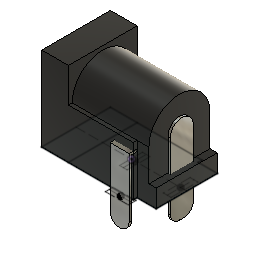
MJ-179PH (Autodesk Fusion 360 design; units mm, degrees)
Autodesk Fusion 360 part; units mm, degrees
sketch "スケッチ1" plane through (0, 0, 0) normal (0, 0, 1) x (1, 0, 0)
  line L0 (-7.25, 4.5) -> (4.75, 4.5)
  line L1 (7.25, 4) -> (7.25, -4)
  line L2 (4.75, -4.5) -> (-7.25, -4.5)
  line L3 (-7.25, -4.5) -> (-7.25, 4.5)
  line L4 (-7.25, 0) -> (7.25, 0) construction
  line L5 (2, -5.4) -> (5, -5.4) construction
  line L6 (5, -5.4) -> (5, -4.4) construction
  line L7 (5, -4.4) -> (2, -4.4) construction
  line L8 (2, -4.4) -> (2, -5.4) construction
  line L9 (-0.05, -1.5) -> (0.95, -1.5) construction
  line L10 (0.95, -1.5) -> (0.95, 1.5) construction
  line L11 (0.95, 1.5) -> (-0.05, 1.5) construction
  line L12 (-0.05, 1.5) -> (-0.05, -1.5) construction
  line L13 (5.95, -1.75) -> (6.95, -1.75) construction
  line L14 (6.95, -1.75) -> (6.95, 1.75) construction
  line L15 (6.95, 1.75) -> (5.95, 1.75) construction
  line L16 (5.95, 1.75) -> (5.95, -1.75) construction
  line L17 (6.45, -1.75) -> (6.45, 1.75) construction
  line L18 (0.45, -1.5) -> (0.45, 1.5) construction
  line L19 (2, -4.9) -> (5, -4.9) construction
  line L20 (4.75, -4.5) -> (4.75, -4)
  line L21 (4.75, -4) -> (7.25, -4)
  line L22 (4.75, 4.5) -> (4.75, 4)
  line L23 (4.75, 4) -> (7.25, 4)
  line L24 (-3.75, -4.5) -> (-3.75, 4.5)
  point P0 (3.5, -4.9)
  point P1 (0.45, 0)
  point P2 (6.45, 0)
  dimension "d2" = 9
  dimension "d3" = 3
  dimension "d4" = 1
  dimension "d5" = 1
  dimension "d6" = 3
  dimension "d7" = 3.5
  dimension "d8" = 1
  dimension "d9" = 7.7
  dimension "d10" = 10.75
  dimension "d11" = 13.7
  dimension "d12" = 4.9
  dimension "d13" = 14.5
  dimension "d14" = 12
  dimension "d15" = 0.5
  dimension "d57" = 3.5
  constraint horizontal L0
  constraint vertical L1
  constraint horizontal L2
  constraint vertical L3
  constraint midpoint L3 L4.start
  constraint midpoint origin L4
  constraint horizontal L5
  constraint vertical L6
  constraint horizontal L7
  constraint vertical L8
  constraint horizontal L9
  constraint vertical L10
  constraint horizontal L11
  constraint vertical L12
  constraint horizontal L13
  constraint vertical L14
  constraint horizontal L15
  constraint vertical L16
  constraint midpoint L13 L17.start
  constraint midpoint L15 L17.end
  constraint midpoint L9 L18.start
  constraint midpoint L11 L18.end
  constraint midpoint L8 L19.start
  constraint midpoint L6 L19.end
  constraint midpoint L19 P0
  constraint midpoint L18 P1
  constraint midpoint L17 P2
  constraint coincident L4 P2
  constraint coincident L4 P1
  constraint perpendicular L2 L20
  constraint perpendicular L1 L21
  constraint perpendicular L0 L22
  constraint perpendicular L1 L23
  constraint coincident L1 L4.end
  constraint midpoint L1 L4.end
  constraint collinear L20 L22
  constraint horizontal L4
  constraint coincident L2 L24.start
  constraint coincident L0 L24.end
  constraint perpendicular L0 L24
  measures "d2" distance of L0.start L2.end
  measures "d3" distance of L5.start L5.end
  measures "d4" distance of L5.start L7.end
  measures "d5" distance of L9.start L9.end
  measures "d6" distance of L9.start L11.end
  measures "d7" distance of L13.end L14.end
  measures "d8" distance of L14.end L15.end
  measures "d9" distance of L3 P1
  measures "d10" distance of L3 P0
  measures "d11" distance of L3 P2
  measures "d12" distance of L4 P0
  measures "d13" distance of L1 L3
  measures "d14" distance of L3 L22
  measures "d15" distance of L0.end L22.end
  measures "d57" distance of L3 L24
sketch "スケッチ3" plane through (0, 0, 0) normal (0, 0, 1) x (1, 0, 0)
  line L0 (2.25, -4.75) -> (4.75, -4.75)
  line L1 (4.75, -4.75) -> (4.75, -5.05)
  line L2 (4.75, -5.05) -> (2.25, -5.05)
  line L3 (2.25, -5.05) -> (2.25, -4.75)
  line L4 (2.25, -4.75) -> (4.75, -5.05) construction
  line L5 (0.3, -1.25) -> (0.3, 1.25)
  line L6 (0.3, 1.25) -> (0.6, 1.25)
  line L7 (0.6, 1.25) -> (0.6, -1.25)
  line L8 (0.6, -1.25) -> (0.3, -1.25)
  line L9 (0.3, 1.25) -> (0.6, -1.25) construction
  line L10 (6.3, -1.5) -> (6.3, 1.5)
  line L11 (6.3, 1.5) -> (6.6, 1.5)
  line L12 (6.6, 1.5) -> (6.6, -1.5)
  line L13 (6.6, -1.5) -> (6.3, -1.5)
  line L14 (6.3, 1.5) -> (6.6, -1.5) construction
  point P0 (3.5, -4.9)
  point P1 (0.45, 0)
  point P2 (6.45, 0)
  dimension "d18" = 2.5
  dimension "d19" = 0.3
  dimension "d20" = 2.5
  dimension "d21" = 0.3
  dimension "d22" = 3
  dimension "d23" = 0.3
  constraint horizontal L0
  constraint vertical L1
  constraint horizontal L2
  constraint vertical L3
  constraint midpoint L4 P0
  constraint midpoint L9 P1
  constraint vertical L5
  constraint horizontal L6
  constraint vertical L7
  constraint horizontal L8
  constraint vertical L10
  constraint horizontal L11
  constraint vertical L12
  constraint horizontal L13
  constraint midpoint L14 P2
  measures "d18" distance of L0.start L0.end
  measures "d19" distance of L0.end L1.end
  measures "d20" distance of L6.end L7.end
  measures "d21" distance of L5.start L7.end
  measures "d22" distance of L11.end L12.end
  measures "d23" distance of L10.start L12.end
sketch "スケッチ5" plane through (0, 0, 0) normal (1, 0, 0) x (0, 1, 0)
  line L0 (4.5, 0) -> (-4.5, 0)
  line L1 (-4.5, 0) -> (-4.5, 11)
  line L2 (-4.5, 11) -> (4.5, 11)
  line L3 (4.5, 11) -> (4.5, 0)
  circle A0 centre (0, 6.5) radius 3
  line L4 (0, 11) -> (0, 0) construction
  circle A1 centre (0, 6.5) radius 0.975
  line L5 (0.975, 6.5) -> (3, 6.5) construction
  circle A2 centre (0, 6.5) radius 1.9875
  line L6 (-1.7319, 5.525) -> (1.7319, 5.525) construction
  point P0 (4.5, 0)
  point P1 (-4.5, 0)
  point P2 (1.9875, 6.5)
  dimension "d26" = 11
  dimension "d27" = 6
  dimension "d28" = 4.5
  dimension "d29" = 9
  dimension "d36" = 1.95
  constraint horizontal L0
  constraint vertical L1
  constraint horizontal L2
  constraint vertical L3
  constraint coincident P0 L0.start
  constraint coincident P1 L0.end
  constraint midpoint L2 L4.start
  constraint coincident L4.end origin
  constraint coincident A0.centre L4
  constraint concentric A0 A1
  constraint coincident A1 L5.start
  constraint coincident A0 L5.end
  constraint horizontal L5
  constraint coincident A0.centre L5
  constraint midpoint L5 P2
  constraint concentric A0 A2
  constraint coincident P2 A2
  constraint coincident A2 L6.start
  constraint coincident A2 L6.end
  constraint perpendicular L4 L6
  constraint tangent A1 L6
  measures "d26" distance of P0 L2.end
  measures "d27" diameter of A0
  measures "d28" distance of L2 A0.centre
  measures "d29" distance of L1.end L2.end
  measures "d36" diameter of A1
sketch "スケッチ4" plane through (0, 0, 0) normal (0, 1, 0) x (1, 0, 0)
  line L0 (-7.25, 0) -> (7.25, 0)
  line L1 (-7.25, 0) -> (-7.25, -11)
  line L2 (-7.25, -11) -> (-3.75, -11)
  line L3 (-3.75, -11) -> (-3.75, -6.5)
  line L4 (-3.75, -6.5) -> (6.3, -6.5)
  line L5 (7.25, 0) -> (7.25, -2.331)
  line L6 (7.25, -2.331) -> (6.3, -2.331)
  line L7 (6.3, -2.331) -> (6.3, -6.5)
  line L8 (4.75, 0) -> (4.75, -6.5)
  line L9 (4.75, -6.5) -> (4.75, -10.5)
  line L10 (4.75, -10.5) -> (-3.75, -10.5)
  line L11 (4.75, -10.5) -> (6.3, -10.5)
  line L12 (6.3, -10.5) -> (6.3, -6.5)
  point P0 (-7.25, 0)
  point P1 (6.3, 0)
  point P2 (4.75, 0)
  point P3 (0, -6.5)
  dimension "d24" = 3.5
  dimension "d25" = 11
  dimension "d30" = 0.5
  constraint coincident P0 L0.start
  constraint perpendicular L0 L1
  constraint perpendicular L1 L2
  constraint perpendicular L2 L3
  constraint perpendicular L3 L4
  constraint coincident L0.end L5.start
  constraint perpendicular L4 L5
  constraint perpendicular L5 L6
  constraint coincident L4 L7.end
  constraint perpendicular L4 L7
  constraint coincident L4.end L7.end
  constraint coincident L7 P1
  constraint coincident P2 L8.start
  constraint coincident L4 L8.end
  constraint perpendicular L4 L8
  constraint coincident L4 P3
  constraint perpendicular L4 L9
  constraint coincident L3 L10.end
  constraint perpendicular L3 L10
  constraint perpendicular L9 L11
  constraint vertical L12
  measures "d24" distance of L1.end L2.end
  measures "d25" distance of P0 L1.end
  measures "d30" distance of L2 L10
extrude "押し出し1" add sketch "スケッチ1" along normal blind 11 makes body 1
extrude "押し出し2" cut sketch "スケッチ4" along normal through all and the other way through all keep common part bodies 1
sketch "スケッチ6" plane through (6.3, 0, 0) normal (1, 0, 0) x (0, 1, 0)
  line L0 (4, 2.331) -> (4, 10.5)
  line L1 (4, 10.5) -> (-4, 10.5)
  line L2 (-4, 10.5) -> (-4, 2.331)
  line L3 (-4, 2.331) -> (4, 2.331)
  arc A0 (4, 6.5) -> (-4, 6.5) centre (0, 6.5) ccw
  line L4 (-4.5, 0) -> (-4.5, 11)
  line L5 (-4, 6.5) -> (-4.5, 6.5)
  line L6 (4.5, 0) -> (4.5, 10.5)
  line L7 (4, 6.5) -> (4.5, 6.5)
  line L8 (-4.5, 0) -> (-4.5, 11)
  line L9 (-4.5, 10.5) -> (-4, 10.5)
  line L10 (-4, 10.5) -> (4, 10.5)
  line L11 (4, 10.5) -> (4.5, 10.5)
  point P0 (0, 6.5)
  point P1 (-4.5, 10.5)
  constraint coincident P0 A0.centre
  constraint tangent L1 A0
  constraint coincident L2 A0.end
  constraint coincident L0 A0.start
  constraint coincident L4 L5.end
  constraint perpendicular L2 L5
  constraint coincident L6 L7.end
  constraint perpendicular L0 L7
extrude "押し出し3" cut sketch "スケッチ6" against normal up to surface (10.05 mm away) contours L0 L1 A0 L10 | L0 L6 L7 L11 | L1 L2 A0 L10 | L2 L4 L5 L8 L9 bodies 1
extrude "押し出し4" add sketch "スケッチ3" against normal blind 3.5 separate body makes body 2 at (3.0833, -4.75, -1.1667) makes body 3 at (6.6, 0.5, -1.1667) makes body 4 at (0.6, 0.4167, -1.1667)
extrude "押し出し5" add sketch "スケッチ3" along normal up to surface (5.525 mm away) contours L0 L1 L2 L3 bodies 2
extrude "押し出し6" add sketch "スケッチ3" along normal up to surface (6.5 mm away) contours L10 L11 L12 L13 bodies 3
sketch "スケッチ7" plane through (6.6, 0, 0) normal (1, 0, 0) x (0, 1, 0)
  line L0 (-1.5, 6.5) -> (-1.5, -3.5)
  line L1 (-1.5, -3.5) -> (1.5, -3.5)
  line L2 (1.5, -3.5) -> (1.5, 6.5)
  line L3 (1.5, 6.5) -> (-1.5, 6.5)
  arc A0 (1.5, 6.5) -> (-1.5, 6.5) centre (0, 6.5) ccw
  point P0 (0, 6.5)
  constraint coincident P0 A0.centre
extrude "押し出し7" add sketch "スケッチ7" against normal up to surface (0.3 mm away) contours L3 A0 bodies 3
sketch "スケッチ8" plane through (0, -5.05, 0) normal (0, -1, 0) x (1, 0, 0)
  line L0 (2.25, 5.525) -> (2.25, -3.5)
  line L1 (2.25, -3.5) -> (4.75, -3.5)
  line L2 (4.75, -3.5) -> (4.75, 5.525)
  line L3 (4.75, 5.525) -> (2.25, 5.525)
  line L4 (2.25, 5.525) -> (4.75, 5.525)
  line L5 (4.75, 5.525) -> (4.75, 5.225)
  line L6 (4.75, 5.225) -> (2.25, 5.225)
  line L7 (2.25, 5.225) -> (2.25, 5.525)
  dimension "d43" = 0.3
  constraint horizontal L4
  constraint vertical L5
  constraint horizontal L6
  constraint vertical L7
  constraint coincident L2 L5.end
  constraint coincident L0.start L3.end
  measures "d43" distance of L0.start L6.end
extrude "押し出し8" add sketch "スケッチ8" against normal blind 1.05 contours L0 L2 L3 L4 L5 L6 L7 bodies 2
extrude "押し出し9" cut sketch "スケッチ5" along normal blind 3.5 and the other way through all contours A0 | A1 | A2 bodies 1
extrude "押し出し10" add sketch "スケッチ5" along normal up to surface (-6.05 mm away) and the other way up to surface (-3.5 mm away) separate body contours A1 makes body 5
fillet "フィレット1" radius 1.25 6 edges at (4.75, -4.9, -3.5) (2.25, -4.9, -3.5) (6.45, -1.5, -3.5) (6.45, 1.5, -3.5) (0.45, -1.25, -3.5) (0.45, 1.25, -3.5) on bodies 2 3 4
fillet "フィレット2" radius 0.9 1 edges at (-6.05, -0.909, 6.1474) on bodies 5
equation "d16 = 6.5 mm + 4.5 mm"
equation "d48 = 0.0 °"
equation "d52 = 0.0 °"
named bodies: "body", "base_pin", "center_pin", "spring_pin", "center"
